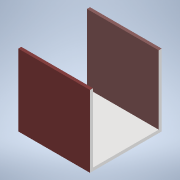
# Autodesk Inventor part: chassisFloor
Saved by Autodesk Inventor 2022.3 (Build 263350000, 350)
## iProperties
Created: 2023-02-06
Part Number: chassisFloor
Material: Generic
Document SubType Name: Modeling
Designer: lbmcgill42
Density: 1 g/cm^3
Appearance: Default
Author: lbmcgill42
Autodesk Inventor part; units mm, degrees
ref_plane "YZ Plane" through (0, 0, 0) normal (1, 0, 0) x (0, 1, 0)
ref_plane "XZ Plane" through (0, 0, 0) normal (0, 1, 0) x (-1, 0, 0)
ref_plane "XY Plane" through (0, 0, 0) normal (0, 0, 1) x (1, 0, 0)
sketch "Sketch1" plane through (0, 0, 0) normal (0, 1, 0) x (-1, 0, 0)
  line L0 (93.0994, 142.6523) -> (-206.6206, 142.6523)
  line L1 (-206.6206, 142.6523) -> (-206.6206, -157.0677)
  line L2 (-206.6206, -157.0677) -> (93.0994, -157.0677)
  line L3 (93.0994, -157.0677) -> (93.0994, 142.6523)
  point P0 (0, 0)
  dimension "d0" = 299.72
  dimension "d1" = 299.72
  constraints: 8 end point, 2 parallel, 1 horizontal, 1 perpendicular
  measures "d0" distance of L2.end L0.start
  measures "d1" distance of L0.start L0.end
extrude "Extrusion1" add sketch "Sketch1" along normal blind 12.7
sketch "Sketch2" plane through (0, 12.7, 0) normal (0, 1, 0) x (1, 0, 0)
  line L0 (-93.0994, -142.6523) -> (206.6206, -142.6523) projected
  line L1 (206.6206, -142.6523) -> (206.6206, 157.0677) projected
  line L2 (-93.0994, -142.6523) -> (206.6206, -142.6523)
  line L3 (206.6206, -142.6523) -> (206.6206, -129.9523)
  line L4 (206.6206, -129.9523) -> (-93.0994, -129.9523)
  line L5 (-93.0994, -129.9523) -> (-93.0994, -142.6523)
  point P0 (0, 0)
  dimension "d4" = 12.7
  constraints: 8 end point, 2 parallel, 1 horizontal, 1 perpendicular, 1 point on line
  measures "d4" distance of L3.end L2.end
extrude "Extrusion2" add sketch "Sketch2" along normal blind 287.02
sketch "Sketch3" plane through (0, 12.7, 0) normal (0, 1, 0) x (1, 0, 0)
  line L0 (-93.0994, 157.0677) -> (-93.0994, -129.9523) projected
  line L1 (206.6206, -129.9523) -> (206.6206, 157.0677) projected
  line L2 (-93.0994, 157.0677) -> (206.6206, 157.0677)
  line L3 (206.6206, 157.0677) -> (206.6206, 144.3677)
  line L4 (206.6206, 144.3677) -> (-93.0994, 144.3677)
  line L5 (-93.0994, 144.3677) -> (-93.0994, 157.0677)
  point P0 (0, 0)
  dimension "d7" = 12.7
  constraints: 8 end point, 2 parallel, 1 horizontal, 1 perpendicular, 1 point on line
  measures "d7" distance of L2.end L3.end
extrude "Extrusion3" add sketch "Sketch3" along normal blind 287.02
body "Solid1"
